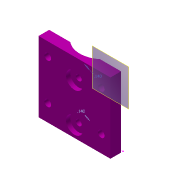
# Autodesk Inventor part: LeadScrewNutCouplerForTrussHeadScrew
Saved by Autodesk Inventor 2018 (Build 220112000, 112)
## iProperties
Created: 2018-12-17
Part Number: LeadScrewNutCouplerForTrussHeadScrew
Material: Generic
Document SubType Name: Modeling
Designer: ball
Density: 1 g/cm^3
Appearance: Default
Author: ball
Autodesk Inventor part; units mm, degrees
ref_plane "YZ Plane" through (0, 0, 0) normal (1, 0, 0) x (0, 1, 0)
ref_plane "XZ Plane" through (0, 0, 0) normal (0, 1, 0) x (-1, 0, 0)
ref_plane "XY Plane" through (0, 0, 0) normal (0, 0, 1) x (1, 0, 0)
ref_plane "Work Plane7" through (21.5, 42.1122, 7.5565) normal (0, 0, -1) x (0, 1, 0)
sketch "Sketch4" plane through (21.5, 42.1122, 7.5565) normal (0, 0, -1) x (0, 1, 0)
  line L0 (-42.1122, -17.69) -> (-42.1122, -25.31) construction
  line L1 (0, 0) -> (0, -43) construction
  line L2 (-528, -43) -> (0, -43) construction
  line L3 (-528, 0) -> (0, 0) construction
  line L4 (-42.1122, -43) -> (0, -43)
  line L5 (0, -43) -> (0, 0)
  line L6 (0, 0) -> (-42.1122, 0)
  line L7 (-42.1122, 0) -> (-42.1122, -43)
  circle A0 centre (-8, -5.5) radius 2
  circle A1 centre (-32, -5.5) radius 2
  circle A2 centre (-8, -37.5) radius 2
  circle A3 centre (-32, -37.5) radius 2
  point P0 (-42.1122, -21.5)
  constraints: 16 end point, 4 centre point, 3 horizontal, 2 parallel, 2 point on line, 2 vertical, 1 perpendicular, 14 other
extrude "Extrusion4" add sketch "Sketch4" along normal blind 6.35
ref_plane "Work Plane6" through (0, 0, 0) normal (0, 0, 1) x (1, 0, 0)
sketch "Sketch5" plane through (0, 0, 0) normal (0, 0, 1) x (1, 0, 0)
  line L0 (3.1132, 0) -> (3.1132, 33.02) construction
  line L1 (-3.1132, 0) -> (-3.1132, 33.02) construction
  line L2 (3.14, 32.92) -> (-3.14, 32.92) construction
  line L3 (-21.5, 0) -> (21.5, 0) construction
  line L4 (3.1132, 0) -> (-3.14, 0)
  line L5 (-3.14, 0) -> (-3.14, 32.92)
  line L6 (-3.14, 32.92) -> (3.1132, 32.92)
  line L7 (3.1132, 32.92) -> (3.1132, 0)
  arc A0 (-0.0115, 8.4836) -> (1.2335, 7.976) centre (0, 6.731) ccw construction
  spline S0 degree 3 poles (-3.9963, 27.1983) (-3.9282, 27.0439) (-3.8705, 26.8672) (-3.7787, 26.4733) (-3.747, 26.2579) (-3.7229, 25.8912) (-3.7161, 25.6578) (-3.7657, 25.2017) (-3.8042, 25.0235) (-3.9064, 24.7384) (-3.9674, 24.6297) (-4.0735, 24.5156) (-4.1125, 24.4855) (-4.225, 24.4328) (-4.3003, 24.4339) (-4.4555, 24.5079) (-4.5339, 24.5853) (-4.6625, 24.7855) (-4.7303, 24.9172) (-4.8354, 25.2648) (-4.8698, 25.4348) (-4.9129, 25.8035) (-4.9196, 25.9997) (-4.906, 26.2838) (-4.8978, 26.3737) (-4.8628, 26.6198) (-4.8272, 26.7652) (-4.7302, 27.0244) (-4.6681, 27.1326) (-4.5976, 27.2088) knots 0 0 0 0 0.142159 0.142159 0.293449 0.293449 0.398535 0.398535 0.47908 0.47908 0.553772 0.553772 0.593008 0.593008 0.662386 0.662386 0.736759 0.736759 0.795223 0.795223 0.84076 0.84076 0.888997 0.888997 0.912398 0.912398 0.954684 0.954684 1 1 1 1 construction
  circle A1 centre (0, 6.731) radius 1.778 construction
  circle A2 centre (-0.0134, 32.92) radius 1.778 construction
  point P0 (0, 0)
  dimension "d10" = 3.556
  dimension "d11" = 3.556
  constraints: 14 end point, 3 centre point, 2 horizontal, 2 parallel, 2 point on circle, 2 vertical, 1 coincident, 1 midpoint, 1 perpendicular, 14 other
  measures "d10" diameter of A1
  measures "d11" diameter of A2
extrude "Extrusion5" add sketch "Sketch5" along normal up to surface (1.2065 mm away)
sketch "Sketch6" plane through (21.5, 42.1122, 7.5565) normal (0, 0, 1) x (1, 0, 0)
  arc A0 (-21.5115, -33.6287) -> (-20.2665, -34.1362) centre (-21.5, -35.3812) ccw construction
  arc A1 (-21.5115, -10.3793) -> (-20.2665, -10.8868) centre (-21.5, -12.1318) ccw construction
  point P0 (-21.5, -42.1122)
  constraints: 4 point on circle, 2 centre point, 8 other
hole "Hole2" at (0, 6.731, 7.5565) at (0, 29.9804, 7.5565) direction (0, 0, -1) diameter 3.556 end through all
ref_plane "Work Plane8" through (21.5, 42.1122, 7.5565) normal (0, 0, 1) x (1, 0, 0)
sketch "Sketch7" plane through (21.5, 42.1122, 7.5565) normal (0, 0, 1) x (1, 0, 0)
  circle A0 centre (-21.5, -12.1318) radius 1.778 projected
  circle A1 centre (-21.5, -12.1318) radius 5.08
  circle A2 centre (-21.5, -35.3812) radius 1.778 projected
  circle A3 centre (-21.5, -35.3812) radius 5.08
  point P0 (-21.5, -42.1122)
  dimension "d28" = 10.16
  dimension "d29" = 10.16
  constraints: 2 centre point, 2 coincident
  measures "d28" diameter of A1
  measures "d29" diameter of A3
extrude "Extrusion6" cut sketch "Sketch7" against normal blind 2.54
sketch "Sketch8" plane through (-21.5, 42.1122, 7.5565) normal (0, 1, 0) x (1, 0, 0)
  circle A0 centre (21.5, 17.145) radius 3.24 construction
  arc A1 (12.6327, 6.35) -> (30.3673, 6.35) centre (21.5, 17.145) ccw
  line L0 (0, 6.35) -> (43, 6.35) projected
  line L1 (12.6327, 6.35) -> (30.3673, 6.35)
  point P0 (21.5, 7.5565)
  dimension "d32" = 27.94
  constraints: 2 centre point, 2 end point, 2 point on circle, 1 coincident, 1 collinear, 1 point on line, 2 other
  measures "d32" diameter of A1
extrude "Extrusion7" cut sketch "Sketch8" against normal blind 9.1948
sketch "Sketch9" plane through (21.5, 42.1122, 1.2065) normal (0, 0, -1) x (-1, 0, 0)
  circle A0 centre (37.5, -8) radius 2 construction
  circle A1 centre (37.5, -8) radius 4.2545 construction
  circle A2 centre (37.5, -32) radius 2 construction
  circle A3 centre (37.5, -32) radius 4.2545 construction
  circle A4 centre (5.5, -8) radius 2 construction
  circle A5 centre (5.5, -8) radius 4.2545 construction
  circle A6 centre (5.5, -32) radius 2 construction
  circle A7 centre (5.5, -32) radius 4.2545 construction
  line L0 (5.5, -12.2545) -> (1.8155, -10.1272)
  line L1 (1.8155, -10.1272) -> (1.8155, -5.8727)
  line L2 (1.8155, -5.8727) -> (5.5, -3.7455)
  line L3 (5.5, -3.7455) -> (9.1845, -5.8727)
  line L4 (9.1845, -5.8727) -> (9.1845, -10.1272)
  line L5 (9.1845, -10.1272) -> (5.5, -12.2545)
  line L6 (5.5, -36.2545) -> (1.8155, -34.1272)
  line L7 (1.8155, -34.1272) -> (1.8155, -29.8727)
  line L8 (1.8155, -29.8727) -> (5.5, -27.7455)
  line L9 (5.5, -27.7455) -> (9.1845, -29.8727)
  line L10 (9.1845, -29.8727) -> (9.1845, -34.1272)
  line L11 (9.1845, -34.1272) -> (5.5, -36.2545)
  line L12 (37.5, -12.2545) -> (33.8155, -10.1272)
  line L13 (33.8155, -10.1272) -> (33.8155, -5.8727)
  line L14 (33.8155, -5.8727) -> (37.5, -3.7455)
  line L15 (37.5, -3.7455) -> (41.1845, -5.8727)
  line L16 (41.1845, -5.8727) -> (41.1845, -10.1272)
  line L17 (41.1845, -10.1272) -> (37.5, -12.2545)
  line L18 (37.5, -36.2545) -> (33.8155, -34.1272)
  line L19 (33.8155, -34.1272) -> (33.8155, -29.8727)
  line L20 (33.8155, -29.8727) -> (37.5, -27.7455)
  line L21 (37.5, -27.7455) -> (41.1845, -29.8727)
  line L22 (41.1845, -29.8727) -> (41.1845, -34.1272)
  line L23 (41.1845, -34.1272) -> (37.5, -36.2545)
  point P0 (21.5, -42.1122)
  dimension "d35" = 8.509
  dimension "d36" = 8.509
  dimension "d37" = 8.509
  dimension "d38" = 8.509
  constraints: 48 end point, 8 coincident, 4 vertical alignment, 60 other
extrude "Extrusion8" cut sketch "Sketch9" against normal blind 1.905
body "Solid2"
